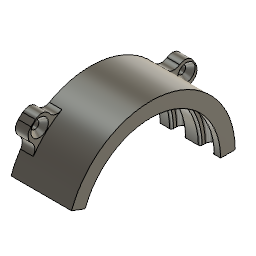
assem_new (Autodesk Fusion 360 archive; units mm, degrees)
design "ring_160"
Autodesk Fusion 360 part; units mm, degrees
note: some values were not read from the file. Chosen so that the rebuilt part matches the saved one: a direction; which face or edge a step refers to. Set by a fixed rule: which sketch regions a step uses.
sketch "Sketch1" plane through (0, 0, 0) normal (0, 0, 1) x (1, 0, 0)
  circle A0 centre (-12.5, 2) radius 1.5
  line L0 (1, -21.5) -> (-17, -21.5)
  line L1 (-17, 0) -> (-17, 5)
  circle A1 centre (-6, 1) radius 1
  line L2 (-17, -21.5) -> (-17, 0)
  line L3 (-14, 2) -> (-14, 1)
  line L4 (-5, 2) -> (-5, 1)
  line L5 (-2, 2) -> (-2, 1)
  circle A2 centre (-15, 1) radius 1
  circle A3 centre (-3.5, 2) radius 1.5
  circle A4 centre (-1, 1) radius 1
  line L6 (1, 0) -> (1, -21.5)
  line L7 (-17, 5) -> (1, 5)
  line L8 (-11, 2) -> (-11, 1)
  line L9 (-17, 0) -> (1, 0)
  circle A5 centre (-10, 1) radius 1
  line L10 (1, 5) -> (1, 0)
  point P0 (-18, 0)
  point P1 (1, 0)
  dimension "d1" = 5
  dimension "d2" = 18
  dimension "d3" = 21.5
  constraint coincident L3.start A0
  constraint coincident L3.end A2
  constraint tangent L3 A2
  constraint coincident L8.start A0
  constraint coincident L8.end A5
  constraint tangent L8 A5
  constraint parallel L3 L8
  constraint coincident L5.start A3
  constraint coincident L5.end A4
  constraint tangent L5 A4
  constraint vertical L5
  constraint coincident L4.start A3
  constraint coincident L4.end A1
  constraint tangent A1 L4
  constraint parallel L4 L5
  constraint horizontal L9
  constraint vertical L6
  constraint horizontal L0
  constraint vertical L2
  measures "d1" distance of L1.start L1.end
  measures "d2" distance of L1.start P1
  measures "d3" distance of L1.start L0.end
revolve "Revolve1" add sketch "Sketch1" angle 160 about axis through (1, -21.5, 0) along (1, 0, 0) contours A0 L1 A1 L3 L4 L5 A2 A3 A4 L7 L8 L9 A5 L10 | A5 | A2 | A1 | A4
move_face "OffsetFaces1" offset -0.2 13 faces at (0.3333, -39.3169, 12.0336) (-1.3717, -38.1094, 13.7645) (-3.0937, -43.9926, 10.7834) (-5.6283, -39.3763, 12.0737) (-7.3333, -39.3169, 12.0336) (-10.3717, -38.1094, 13.7645) (-12.0937, 3.414, 1.2216) (-14.6283, -39.3763, 12.0737) (-16.3333, -41.319, 8.334) (-14, -38.5613, 15.5889) (-5, -18.0303, 22.8488) (-11, -18.0303, 22.8488) (-2, -18.0303, 22.8488)
move_face "OffsetFaces2" offset -0.2 13 faces at (-10.8, -18.0303, 22.8488) (-12.9604, -42.9944, 13.0319) (-10.2973, -41.1191, 9.4058) (-14.2, -42.3462, 9.977) (-7.3333, -41.5034, 8.4115) (-14.7027, -23.5621, 21.6594) (-16.3333, -4.7072, 13.7439) (-0.3333, 0.0959, 2.1228) (-1.2973, -41.1191, 9.4058) (-1.8, -18.0303, 22.8488) (-3.9604, -42.9944, 13.0319) (-5.2, -18.0303, 22.8488) (-5.7027, -11.2033, 19.1666)
sketch "Sketch2" plane through (-17, 0, 0) normal (-1, 0, 0) x (0, -1, 0)
  line L0 (-5, 0) -> (-0.4, 0)
  arc A0 (42.0793, 7.4902) -> (-0.4, 0) centre (21.5, 0) ccw
  line L1 (42.0793, 7.4902) -> (46.4019, 9.0635)
  arc A1 (46.4019, 9.0635) -> (-5, 0) centre (21.5, 0) ccw
  circle A2 centre (21.5, 0) radius 32.5
  line L2 (21.5, 0) -> (-9.04, 11.1157)
  line L3 (21.5, 0) -> (54, 0) construction
  line L4 (21.5, 0) -> (-5.1224, 18.6412)
  line L5 (21.5, 0) -> (54, 0) construction
  line L6 (21.5, 0) -> (-4.6668, 13.6216)
  line L7 (21.5, 0) -> (51, 0) construction
  line L8 (21.5, 0) -> (46.3964, 20.8906)
  line L9 (21.5, 0) -> (54, 0) construction
  line L10 (21.5, 0) -> (40.1412, 26.6224)
  line L11 (21.5, 0) -> (54, 0) construction
  line L12 (21.5, 0) -> (41.4299, 21.7497)
  line L13 (21.5, 0) -> (51, 0) construction
  circle A3 centre (-4.6668, 13.6216) radius 1.25
  circle A4 centre (41.4299, 21.7497) radius 1.25
  dimension "d7" = 65
  dimension "d8" = 160
  dimension "d9" = 145
  dimension "d10" = 152.5
  dimension "d11" = 29.5
  dimension "d12" = 40
  dimension "d13" = 55
  dimension "d14" = 47.5
  dimension "d15" = 29.5
  dimension "d16" = 2.5
  dimension "d17" = 2.5
  dimension "d18" = 32.5
  constraint concentric A0 A2
  constraint horizontal L3
  constraint coincident A0.centre A1.centre
  constraint horizontal L5
  constraint horizontal L7
  constraint horizontal L9
  constraint horizontal L11
  constraint horizontal L13
  constraint coincident L6.end A3.centre
  constraint coincident L12.end A4.centre
  measures "d7" diameter of A2
  measures "d8" angle of L2 L3
  measures "d9" angle of L4 L5
  measures "d10" angle of L6 L7
  measures "d11" distance of A0.centre L6.end
  measures "d12" angle of L8 L9
  measures "d13" angle of L10 L11
  measures "d14" angle of L12 L13
  measures "d15" distance of A0.centre L12.end
  measures "d16" diameter of A3
  measures "d17" diameter of A4
  measures "d18" distance of A0.centre L4.end
extrude "Extrude1" add sketch "Sketch2" against normal blind 3 contours A1 A2 L2 L4 | A1 A2 L8 L10
extrude "Extrude2" add 1 faces at (-17, 0.6845, 12.5418) along direction (-1, 0, 0) blind 1
fillet "Fillet1" radius 3 8 edges at (-16, 0.2075, 15.1998) (-16, 5.1224, 18.6412) (-16, 9.04, 11.1157) (-16, 3.4019, 9.0635) (-16, -36.6998, 21.7075) (-16, -40.1412, 26.6224) (-16, -41.8002, 17.0339) (-16, -46.3964, 20.8906)
chamfer "Chamfer1" distance 1.5 angle 45 2 edges at (-14, 5.8322, 13.1696) (-14, -40.2645, 21.2977)

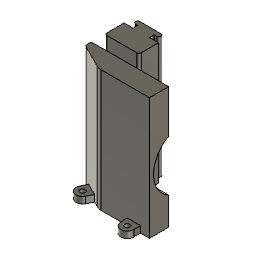
design "vertical_servo_mount"
Autodesk Fusion 360 part; units mm, degrees
sketch "Sketch1" plane through (0, 0, 0) normal (0, 0, 1) x (1, 0, 0)
  line L0 (0, 0) -> (35, 0)
  line L1 (35, 0) -> (35, -25)
  line L2 (35, -25) -> (0, -25)
  line L3 (0, -25) -> (0, 0)
  dimension "d1" = 35
  dimension "d2" = 25
  constraint horizontal L0
  constraint vertical L1
  constraint horizontal L2
  constraint vertical L3
  constraint coincident L0.start L3.end
  measures "d1" distance of L0.start L0.end
  measures "d2" distance of L0.start L2.end
extrude "Extrude1" add sketch "Sketch1" along normal blind 55
sketch "Sketch2" plane through (0, 0, 0) normal (0, 1, 0) x (-1, 0, 0)
  line L0 (-35, 0) -> (0, 0)
  line L1 (0, 0) -> (0, 55)
  line L2 (0, 55) -> (-35, 55)
  line L3 (-35, 55) -> (-35, 0)
  line L4 (-22.7083, 24.0993) -> (-22.7083, 25.6362)
  line L5 (-5.5083, 17.9993) -> (-15.8083, 17.9993)
  line L6 (-5.5083, 18.8493) -> (-0.2083, 18.8493)
  line L7 (-5.5083, 17.9993) -> (-5.5083, 18.8493)
  line L8 (-26.7583, 17.9993) -> (-26.7583, 29.4909)
  line L9 (-15.8083, 14.0493) -> (-15.8083, 13.1993)
  line L10 (-22.7083, 24.0993) -> (-22.7083, 25.6362)
  line L11 (-31.7583, 25.9993) -> (-31.7583, 22.1993)
  line L12 (-15.8083, 44.4493) -> (-15.8083, 14.0493)
  line L13 (-18.3083, 17.9993) -> (-22.5083, 17.9993)
  line L14 (-0.2083, 39.6493) -> (-0.2083, 18.8493)
  line L15 (-15.8083, 18.8493) -> (-15.8083, 17.9993)
  line L16 (-5.5083, 39.6493) -> (-5.5083, 18.8493)
  line L17 (-5.5083, 18.8493) -> (-5.5083, 17.9993)
  line L18 (-30.3583, 22.1993) -> (-30.3583, 25.9993)
  line L19 (-18.3083, 18.8493) -> (-22.5083, 18.8493)
  line L20 (-15.8083, 18.8493) -> (-15.8083, 39.6493)
  line L21 (-15.8083, 14.0493) -> (-18.3083, 14.0493)
  line L22 (-31.7583, 27.5493) -> (-31.7583, 21.8903)
  line L23 (-18.3083, 14.0493) -> (-18.3083, 18.8493)
  line L24 (-0.2083, 17.9993) -> (-5.5083, 17.9993)
  line L25 (-27.9583, 27.5493) -> (-27.9583, 20.6493)
  line L26 (-15.8083, 18.8493) -> (-5.5083, 18.8493)
  line L27 (-5.5083, 18.8493) -> (-5.5083, 39.6493)
  line L28 (-5.5083, 40.4993) -> (-5.5083, 39.6493)
  line L29 (-22.7083, 29.4909) -> (-26.7583, 29.4909)
  line L30 (-0.2083, 39.6493) -> (-5.5083, 39.6493)
  line L31 (-5.5083, 39.6493) -> (-5.5083, 40.4993)
  line L32 (-30.3583, 9.9402) -> (-31.7583, 9.9402)
  line L33 (-31.7583, 40.7256) -> (-30.3583, 40.7256)
  line L34 (-31.7583, 9.9402) -> (-31.7583, 8.0493)
  line L35 (-18.3083, 45.2993) -> (-18.3083, 44.4493)
  line L36 (-22.7083, 22.5625) -> (-22.7083, 24.0993)
  line L37 (-22.7083, 22.5625) -> (-22.7083, 18.1961)
  line L38 (-31.7583, 22.1993) -> (-30.3583, 22.1993)
  line L39 (-31.7583, 25.9993) -> (-30.3583, 25.9993)
  line L40 (-26.7583, 29.4909) -> (-22.7083, 29.4909)
  line L41 (-22.7083, 22.5625) -> (-22.7083, 18.1961)
  line L42 (-22.7083, 17.9993) -> (-22.7083, 18.1961)
  line L43 (-31.7583, 9.9402) -> (-30.3583, 9.9402)
  line L44 (-31.7583, 21.8903) -> (-30.3583, 21.8903)
  line L45 (-31.7583, 25.9993) -> (-31.7583, 40.7256)
  line L46 (-26.7583, 29.6993) -> (-26.7583, 32.4993)
  line L47 (-15.8083, 40.4993) -> (-5.5083, 40.4993)
  line L48 (-30.3583, 22.1993) -> (-31.7583, 22.1993)
  line L49 (-30.3583, 40.7256) -> (-30.3583, 25.9993)
  line L50 (-30.3583, 25.9993) -> (-30.3583, 40.7256)
  line L51 (-31.7583, 40.7256) -> (-31.7583, 25.9993)
  line L52 (-18.3083, 45.2993) -> (-15.8083, 45.2993)
  line L53 (-5.5083, 39.6493) -> (-0.2083, 39.6493)
  line L54 (-18.3083, 39.6493) -> (-18.3083, 44.4493)
  line L55 (-22.7083, 29.4909) -> (-22.7083, 25.6362)
  line L56 (-0.2083, 18.8493) -> (-5.5083, 18.8493)
  line L57 (-18.3083, 18.8493) -> (-18.3083, 17.9993)
  line L58 (-18.3083, 14.0493) -> (-18.3083, 13.1993)
  line L59 (-15.8083, 13.1993) -> (-18.3083, 13.1993)
  line L60 (-22.5083, 18.8493) -> (-22.5083, 22.5373)
  line L61 (-15.8083, 44.4493) -> (-18.3083, 44.4493)
  line L62 (-22.7083, 22.5625) -> (-22.7083, 24.0993)
  line L63 (-22.7083, 17.9993) -> (-22.7083, 18.1961)
  line L64 (-31.7583, 9.9402) -> (-31.7583, 21.8903)
  line L65 (-22.5083, 25.6614) -> (-22.5083, 39.6493)
  line L66 (-30.3583, 21.8903) -> (-31.7583, 21.8903)
  line L67 (-30.3583, 20.6493) -> (-30.3583, 21.8903)
  line L68 (-22.5083, 40.4993) -> (-18.3083, 40.4993)
  line L69 (-0.2083, 40.4993) -> (-0.2083, 39.6493)
  line L70 (-15.8083, 39.6493) -> (-5.5083, 39.6493)
  line L71 (-5.5083, 40.4993) -> (-0.2083, 40.4993)
  line L72 (-15.8083, 40.4993) -> (-15.8083, 39.6493)
  line L73 (-30.3583, 9.9402) -> (-30.3583, 8.0493)
  line L74 (-30.3583, 40.7256) -> (-30.3583, 42.5493)
  line L75 (-15.8083, 45.2993) -> (-15.8083, 44.4493)
  line L76 (-18.3083, 44.4493) -> (-15.8083, 44.4493)
  line L77 (-22.7083, 29.4909) -> (-22.7083, 25.6362)
  line L78 (-5.5083, 39.6493) -> (-15.8083, 39.6493)
  line L79 (-31.7583, 21.8903) -> (-30.3583, 21.8903)
  line L80 (-30.3583, 22.1993) -> (-31.7583, 22.1993)
  line L81 (-31.7583, 25.9993) -> (-30.3583, 25.9993)
  line L82 (-18.3083, 40.4993) -> (-18.3083, 39.6493)
  line L83 (-30.3583, 25.9993) -> (-31.7583, 25.9993)
  line L84 (-22.5083, 17.9993) -> (-22.5083, 18.8493)
  line L85 (-30.3583, 21.8903) -> (-30.3583, 9.9402)
  line L86 (-22.5083, 22.5373) -> (-22.5083, 24.0993)
  line L87 (-22.7083, 32.4993) -> (-22.7083, 29.6993)
  line L88 (-22.7083, 29.6993) -> (-26.7583, 29.6993)
  line L89 (-31.7583, 40.7256) -> (-30.3583, 40.7256)
  line L90 (-22.5083, 39.6493) -> (-22.5083, 40.4993)
  line L91 (-30.3583, 25.9993) -> (-31.7583, 25.9993)
  line L92 (-26.7583, 29.6993) -> (-22.7083, 29.6993)
  line L93 (-22.5083, 39.6493) -> (-18.3083, 39.6493)
  line L94 (-18.3083, 39.6493) -> (-22.5083, 39.6493)
  line L95 (-0.2083, 18.8493) -> (-0.2083, 17.9993)
  line L96 (-30.3583, 9.9402) -> (-31.7583, 9.9402)
  line L97 (-30.3583, 21.8903) -> (-30.3583, 9.9402)
  line L98 (-31.7583, 42.5493) -> (-31.7583, 40.7256)
  line L99 (-30.3583, 40.7256) -> (-31.7583, 40.7256)
  line L100 (-22.5083, 18.8493) -> (-18.3083, 18.8493)
  line L101 (-18.3083, 14.0493) -> (-15.8083, 14.0493)
  line L102 (-5.5083, 18.8493) -> (-15.8083, 18.8493)
  line L103 (-22.5083, 24.0993) -> (-22.5083, 25.6614)
  line L104 (-0.2083, 40.4993) -> (0, 40.4993)
  line L105 (-0.2083, 17.9993) -> (0, 17.9993)
  line L106 (0, 40.4993) -> (-15.6, 40.4993)
  line L107 (-15.6, 40.4993) -> (-15.6, 46.4993)
  line L108 (-15.6, 46.4993) -> (0, 46.4993)
  line L109 (0, 46.4993) -> (0, 40.4993)
  line L110 (0, 17.9993) -> (-15.6, 17.9993)
  line L111 (-15.6, 17.9993) -> (-15.6, 11.9993)
  line L112 (-15.6, 11.9993) -> (0, 11.9993)
  line L113 (0, 11.9993) -> (0, 17.9993)
  line L114 (-15.6, 46.4993) -> (-15.6, 55)
  line L115 (-15.6, 11.9993) -> (-15.6, 0)
  dimension "d5" = 15.6
  dimension "d6" = 6
  dimension "d7" = 15.6
  dimension "d8" = 6
  constraint coincident L1 L104.end
  constraint perpendicular L1 L104
  constraint coincident L1 L105.end
  constraint perpendicular L1 L105
  constraint horizontal L106
  constraint vertical L107
  constraint horizontal L108
  constraint vertical L109
  constraint horizontal L110
  constraint vertical L111
  constraint horizontal L112
  constraint vertical L113
  constraint coincident L2 L114.end
  constraint perpendicular L2 L114
  constraint coincident L0 L115.end
  constraint perpendicular L0 L115
  measures "d5" distance of L104.end L106.end
  measures "d6" distance of L104.end L108.end
  measures "d7" distance of L105.end L110.end
  measures "d8" distance of L105.end L112.end
extrude "Extrude2" cut sketch "Sketch2" against normal blind 12.2 contours L0 L2 L3 L5 L9 L12 L13 L23 L35 L47 L52 L54 L58 L59 L60 L65 L68 L75 L84 L86 L90 L103 L107 L111 L114 L115 | L5 L7 L12 L15 L17 L26 L102 L110 | L1 L14 L69 L95 L104 L105 L106 L110 | L6 L7 L17 L24 L56 L95 L110 | L12 L15 L19 L20 L21 L23 L54 L57 L60 L61 L65 L72 L76 L82 L86 L93 L94 L100 L101 L103 | L6 L14 L16 L27 L30 L53 L56 | L12 L16 L20 L26 L27 L70 L78 L102 | L9 L21 L58 L59 L101 | L35 L52 L61 L75 L76 | L13 L19 L23 L57 L84 L100 | L54 L68 L82 L90 L93 L94 | L11 L18 L22 L38 L39 L48 L80 L81 L83 L91 | L22 L33 L39 L45 L49 L50 L51 L81 L83 L89 L91 L99 | L32 L43 L44 L64 L66 L67 L79 L85 L96 L97
extrude "Extrude3" cut sketch "Sketch2" against normal blind 12.2 contours L12 L28 L31 L47 L70 L72 L78 L106 | L28 L30 L31 L53 L69 L71 L106
sketch "Sketch3" plane through (15.6, 0, 0) normal (1, 0, 0) x (0, 1, 0)
  line L0 (0, 40.4993) -> (0, 55)
  line L1 (0, 55) -> (-12.2, 55)
  line L2 (-12.2, 55) -> (-12.2, 40.4993)
  line L3 (-12.2, 40.4993) -> (0, 40.4993)
  line L4 (-12.2, 40.4993) -> (-6.1, 40.4993)
  line L5 (-6.1, 40.4993) -> (-6.1, 43.1493)
  circle A0 centre (-6.1, 43.1493) radius 0.75
  dimension "d13" = 2.65
  dimension "d14" = 1.5
  constraint coincident L2.end L3.start
  constraint midpoint L3 L4.end
  constraint perpendicular L4 L5
  constraint coincident L5.end A0.centre
  measures "d13" distance of L4.end L5.end
  measures "d14" diameter of A0
extrude "Extrude4" cut sketch "Sketch3" against normal blind 5 contours A0
sketch "Sketch4" plane through (15.6, 0, 0) normal (1, 0, 0) x (0, 1, 0)
  line L0 (0, 0) -> (0, 17.9993)
  line L1 (0, 17.9993) -> (-12.2, 17.9993)
  line L2 (-12.2, 17.9993) -> (-12.2, 0)
  line L3 (-12.2, 0) -> (0, 0)
  line L4 (-12.2, 17.9993) -> (-6.1, 17.9993)
  line L5 (-6.1, 17.9993) -> (-6.1, 15.3493)
  circle A0 centre (-6.1, 15.3493) radius 0.75
  dimension "d17" = 2.65
  dimension "d18" = 1.5
  constraint coincident L1.end L2.start
  constraint midpoint L1 L4.end
  constraint perpendicular L4 L5
  constraint coincident L5.end A0.centre
  measures "d17" distance of L4.end L5.end
  measures "d18" diameter of A0
extrude "Extrude5" cut sketch "Sketch4" against normal blind 5 contours A0
move_face "OffsetFaces1" offset -0.2 1 faces at (5.2, -8.1333, 17.9993)
move_face "OffsetFaces2" offset -0.2 1 faces at (10.4, -8.1333, 40.4993)
move_face "OffsetFaces3" offset -0.1 1 faces at (28.5333, -12.2, 24.2664)
sketch "Sketch5" plane through (15.6, 0, 0) normal (1, 0, 0) x (0, 1, 0)
  circle A0 centre (-6.1, 43.1493) radius 0.75
  line L0 (0, 40.6993) -> (0, 55)
  line L1 (0, 55) -> (-12.3, 55)
  line L2 (-12.3, 55) -> (-12.3, 40.6993)
  line L3 (-12.3, 40.6993) -> (0, 40.6993)
  line L4 (-6.15, 40.6993) -> (-6.15, 17.9993)
  line L5 (-6.15, 40.6993) -> (-6.15, 40.4993)
  line L6 (-6.15, 40.4993) -> (-6.15, 24.0993)
  circle A1 centre (-6.15, 24.0993) radius 12.5
  dimension "d24" = 22.7
  dimension "d25" = 0.2
  dimension "d26" = 16.4
  dimension "d27" = 25
  constraint midpoint L3 L4.start
  constraint perpendicular L3 L4
  constraint perpendicular L3 L5
  constraint parallel L4 L6
  constraint coincident L6.end A1.centre
  measures "d24" distance of L4.start L4.end
  measures "d25" distance of L4.start L5.end
  measures "d26" distance of L5.end L6.end
  measures "d27" diameter of A1
extrude "Extrude6" cut sketch "Sketch5" along normal blind 32 contours A1
move_face "OffsetFaces4" offset -0.5 1 faces at (28.5333, -13.2933, 34.3572)
move_face "OffsetFaces5" offset -4 1 faces at (23.3333, -25, 36.6667)
sketch "Sketch6" plane through (0, 0, 0) normal (0, 1, 0) x (-1, 0, 0)
  line L0 (-15.6, 40.6993) -> (0, 40.6993)
  line L1 (0, 40.6993) -> (0, 55)
  line L2 (0, 55) -> (-15.6, 55)
  line L3 (-15.6, 55) -> (-15.6, 40.6993)
  line L4 (-15.6, 55) -> (0, 55)
  line L5 (0, 55) -> (0, 0)
  line L6 (0, 0) -> (-15.6, 0)
  line L7 (-15.6, 0) -> (-15.6, 55)
  constraint horizontal L4
  constraint vertical L5
  constraint horizontal L6
  constraint vertical L7
  constraint coincident L5.end L6.start
  constraint coincident L2.end L3.start
extrude "Extrude7" add sketch "Sketch6" along normal blind 6.652
move_face "OffsetFaces6" offset -0.1 1 faces at (10.4, 0, 25.4327)
sketch "Sketch7" plane through (0, 0, 0) normal (-1, 0, 0) x (0, -1, 0)
  line L0 (-0.1, 40.6993) -> (12.3, 40.6993)
  line L1 (12.3, 40.6993) -> (12.3, 17.7993)
  line L2 (12.3, 17.7993) -> (-0.1, 17.7993)
  line L3 (-0.1, 17.7993) -> (-0.1, 40.6993)
  line L4 (21, 55) -> (-6.652, 55)
  line L5 (-6.652, 55) -> (-6.652, 0)
  line L6 (-6.652, 0) -> (21, 0)
  line L7 (21, 0) -> (21, 55)
  line L8 (-6.652, 0) -> (-2.552, 0)
  line L9 (-2.552, 0) -> (-2.552, 55)
  line L10 (-2.552, 55) -> (-6.652, 55)
  line L11 (-6.652, 55) -> (-6.652, 0)
  line L12 (-2.552, 55) -> (-4.652, 55)
  line L13 (-4.652, 55) -> (-4.652, 0)
  line L14 (-4.652, 0) -> (-2.552, 0)
  line L15 (-2.552, 0) -> (-2.552, 55)
  dimension "d35" = 4.1
  dimension "d36" = 2.1
  constraint horizontal L8
  constraint vertical L9
  constraint horizontal L10
  constraint vertical L11
  constraint coincident L5.end L6.start
  constraint horizontal L12
  constraint vertical L13
  constraint horizontal L14
  constraint vertical L15
  measures "d35" distance of L5.end L8.end
  measures "d36" distance of L9.end L12.end
extrude "Extrude8" cut sketch "Sketch7" against normal blind 2 contours L4 L5 L6 L8 L10 L11 L13
extrude "Extrude9" cut sketch "Sketch7" against normal blind 4 contours L4 L6 L8 L9 L10 L12 L13 L14 L15
sketch "Sketch8" plane through (15.6, 0, 0) normal (1, 0, 0) x (0, 1, 0)
  circle A0 centre (-6.1, 15.3493) radius 0.75
  circle A1 centre (-6.1, 43.1493) radius 0.75
  line L0 (6.652, 55) -> (-12.3, 55)
  line L1 (-12.3, 55) -> (-12.3, 40.6993)
  line L2 (-12.3, 40.6993) -> (0.1, 40.6993)
  line L3 (0.1, 40.6993) -> (0.1, 17.7993)
  line L4 (0.1, 17.7993) -> (-12.3, 17.7993)
  line L5 (-12.3, 17.7993) -> (-12.3, 35.5526)
  arc A2 (-12.3, 35.5526) -> (-12.3, 12.6461) centre (-6.15, 24.0993) ccw
  line L6 (-12.3, 12.6461) -> (-12.3, 0)
  line L7 (-12.3, 0) -> (6.652, 0)
  line L8 (6.652, 0) -> (6.652, 55)
  line L9 (6.652, 55) -> (2.552, 55)
  line L10 (2.552, 55) -> (2.552, 0)
  line L11 (2.552, 0) -> (6.652, 0)
  line L12 (6.652, 0) -> (6.652, 55)
  line L13 (6.652, 55) -> (4.652, 55)
  line L14 (4.652, 55) -> (4.652, 0)
  line L15 (4.652, 0) -> (6.652, 0)
  line L16 (6.652, 0) -> (6.652, 55)
  dimension "d41" = 4.1
  dimension "d42" = 2
  constraint horizontal L9
  constraint vertical L10
  constraint horizontal L11
  constraint vertical L12
  constraint coincident L0.start L8.end
  constraint horizontal L13
  constraint vertical L14
  constraint horizontal L15
  constraint vertical L16
  measures "d41" distance of L0.start L9.end
  measures "d42" distance of L0.start L13.end
extrude "Extrude10" cut sketch "Sketch8" against normal blind 2 contours L0 L7 L8 L9 L11 L12 L13 L14 L15 L16
extrude "Extrude11" cut sketch "Sketch8" against normal blind 4 contours L0 L7 L9 L10 L11 L14
fillet "Fillet1" radius 1 4 edges at (2, 4.652, 27.5) (2, 6.652, 27.5) (13.6, 4.652, 27.5) (13.6, 6.652, 27.5)
sketch "Sketch9" plane through (0, 0, 0) normal (-1, 0, 0) x (0, -1, 0)
  line L0 (-2.552, 55) -> (-2.552, 0)
  line L1 (-2.552, 0) -> (21, 0)
  line L2 (21, 0) -> (21, 55)
  line L3 (21, 55) -> (-2.552, 55)
  line L4 (-0.1, 40.6993) -> (12.3, 40.6993)
  line L5 (12.3, 40.6993) -> (12.3, 17.7993)
  line L6 (12.3, 17.7993) -> (-0.1, 17.7993)
  line L7 (-0.1, 17.7993) -> (-0.1, 40.6993)
  line L8 (6.1, 17.7993) -> (6.1, 10.7993)
  line L9 (6.1, 10.7993) -> (11.1, 10.7993)
  line L10 (11.1, 10.7993) -> (11.1, 17.7993)
  line L11 (11.1, 17.7993) -> (6.1, 17.7993)
  line L12 (6.1, 17.7993) -> (6.1, 10.7993)
  line L13 (6.1, 10.7993) -> (1.1, 10.7993)
  line L14 (1.1, 10.7993) -> (1.1, 17.7993)
  line L15 (1.1, 17.7993) -> (6.1, 17.7993)
  line L16 (6.1, 17.7993) -> (6.1, 10.7993)
  line L17 (6.1, 17.7993) -> (9.1, 17.7993)
  line L18 (9.1, 17.7993) -> (9.1, 16.7993)
  line L19 (9.1, 16.7993) -> (6.1, 16.7993)
  line L20 (6.1, 16.7993) -> (6.1, 17.7993)
  line L21 (6.1, 16.7993) -> (3.1, 16.7993)
  line L22 (3.1, 16.7993) -> (3.1, 17.7993)
  line L23 (3.1, 17.7993) -> (6.1, 17.7993)
  line L24 (6.1, 17.7993) -> (6.1, 16.7993)
  dimension "d49" = 7
  dimension "d50" = 5
  dimension "d51" = 7
  dimension "d52" = 3
  dimension "d53" = 1
  dimension "d54" = 3
  constraint midpoint L6 L8.start
  constraint perpendicular L6 L8
  constraint horizontal L9
  constraint vertical L10
  constraint horizontal L11
  constraint vertical L12
  constraint horizontal L13
  constraint vertical L14
  constraint horizontal L15
  constraint vertical L16
  constraint horizontal L17
  constraint vertical L18
  constraint horizontal L19
  constraint vertical L20
  constraint horizontal L21
  constraint vertical L22
  constraint horizontal L23
  constraint vertical L24
  measures "d49" distance of L8.start L8.end
  measures "d50" distance of L8.end L9.end
  measures "d51" distance of L8.end L8.start
  measures "d52" distance of L8.start L17.end
  measures "d53" distance of L8.start L19.end
  measures "d54" distance of L19.end L21.end
extrude "Extrude12" cut sketch "Sketch9" against normal blind 10 contours L6 L8 L12 L13 L14 L15 L16 L21 L22 | L6 L8 L9 L10 L11 L12 L16 L18 L19
extrude "Extrude13" cut 1 faces at (0, -7.1, 17.1327) along direction (1, 0, 0) blind 10
extrude "Extrude14" cut sketch "Sketch9" against normal blind 23 contours L6 L8 L12 L15 L16 L20 L21 L22 L23 L24 | L6 L8 L11 L12 L16 L17 L18 L19 L20 L24
fillet "Fillet2" radius 1 4 edges at (12.8, -3.1, 16.7993) (12.8, -3.1, 17.7993) (12.8, -9.1, 17.7993) (12.8, -9.1, 16.7993)
move_face "OffsetFaces7" offset -0.1 2 faces at (11.6, 3.252, 18.3333) (4, 3.952, 18.3333)
sketch "Sketch10" plane through (0, 0, 55) normal (0, 0, 1) x (-1, 0, 0)
  arc A0 (-12.6, -4.652) -> (-12.6, -6.652) centre (-12.6, -5.652) ccw
  line L0 (-12.6, -6.652) -> (-3, -6.652)
  arc A1 (-3, -6.652) -> (-3, -4.652) centre (-3, -5.652) ccw
  line L1 (-3, -4.652) -> (-4.1, -4.652)
  line L2 (-4.1, -4.652) -> (-4.1, -2.552)
  line L3 (-4.1, -2.552) -> (0, -2.552)
  line L4 (0, -2.552) -> (0, 21)
  line L5 (0, 21) -> (-35, 21)
  line L6 (-35, 21) -> (-35, 12.3)
  line L7 (-35, 12.3) -> (-15.6, 12.3)
  line L8 (-15.6, 12.3) -> (-15.6, -2.552)
  line L9 (-15.6, -2.552) -> (-11.5, -2.552)
  line L10 (-11.5, -2.552) -> (-11.5, -4.652)
  line L11 (-11.5, -4.652) -> (-12.6, -4.652)
  line L12 (-15.6, 12.3) -> (0, 12.3)
  line L13 (0, 12.3) -> (0, 6.3)
  line L14 (0, 6.3) -> (-15.6, 6.3)
  line L15 (-15.6, 6.3) -> (-15.6, 12.3)
  dimension "d64" = 6
  constraint horizontal L12
  constraint vertical L13
  constraint horizontal L14
  constraint vertical L15
  constraint coincident L7.end L8.start
  measures "d64" distance of L7.end L14.end
extrude "Extrude15" cut sketch "Sketch10" against normal blind 10 contours L4 L8 L12 L13 L14 L15
fillet "Fillet3" radius 1 5 edges at (15.6, -9.3, 45) (15.6, -6.3, 50) (0, -12.3, 50) (0, -6.3, 50) (0, -9.3, 45)
sketch "Sketch11" plane through (0, 0, 55) normal (0, 0, 1) x (-1, 0, 0)
  arc A0 (-1, 12.3) -> (0, 13.3) centre (-1, 13.3) ccw
  line L0 (0, 13.3) -> (0, 21)
  line L1 (0, 21) -> (-35, 21)
  line L2 (-35, 21) -> (-35, 12.3)
  line L3 (-35, 12.3) -> (-1, 12.3)
  line L4 (0, 21) -> (0, 15)
  line L5 (0, 21) -> (-12, 21)
  line L6 (0, 15) -> (-12, 21)
  dimension "d69" = 12
  constraint coincident L0.end L1.start
  constraint coincident L0 L4.end
  constraint perpendicular L4 L5
  measures "d69" distance of L0.end L5.end
extrude "Extrude16" cut sketch "Sketch11" against normal blind 100 contours L0 L1 L4 L5 L6
fillet "Fillet4" radius 1.5 1 edges at (0, -15, 27.5)
fillet "Fillet5" radius 5 1 edges at (12, -21, 27.5)
sketch "Sketch12" plane through (0, 0, 0) normal (0, 0, -1) x (1, 0, 0)
  arc A0 (13.1803, 21) -> (10.9443, 20.4721) centre (13.1803, 16) ccw
  line L0 (10.9443, 20.4721) -> (0.8292, 15.4146)
  arc A1 (0.8292, 15.4146) -> (0, 14.0729) centre (1.5, 14.0729) ccw
  line L1 (0, 14.0729) -> (0, -2.552)
  line L2 (0, -2.552) -> (4.1, -2.552)
  line L3 (4.1, -2.552) -> (4.1, -4.652)
  line L4 (4.1, -4.652) -> (3, -4.652)
  arc A2 (3, -4.652) -> (3, -6.652) centre (3, -5.652) ccw
  line L5 (3, -6.652) -> (12.6, -6.652)
  arc A3 (12.6, -6.652) -> (12.6, -4.652) centre (12.6, -5.652) ccw
  line L6 (12.6, -4.652) -> (11.5, -4.652)
  line L7 (11.5, -4.652) -> (11.5, -2.552)
  line L8 (11.5, -2.552) -> (15.6, -2.552)
  line L9 (15.6, -2.552) -> (15.6, 12.3)
  line L10 (15.6, 12.3) -> (35, 12.3)
  line L11 (35, 12.3) -> (35, 21)
  line L12 (35, 21) -> (13.1803, 21)
  line L13 (35, 21) -> (31, 21)
  line L14 (31, 21) -> (25, 21)
  line L15 (25, 21) -> (25, 27)
  line L16 (25, 27) -> (31, 27)
  line L17 (31, 27) -> (31, 21)
  circle A4 centre (28, 24) radius 1.15
  circle A5 centre (28, 24) radius 3
  line L18 (0, -2.552) -> (0, 1.448)
  line L19 (0, 1.448) -> (-6, 1.448)
  line L20 (-6, 1.448) -> (-6, 7.448)
  line L21 (-6, 7.448) -> (0, 7.448)
  line L22 (0, 7.448) -> (0, 1.448)
  circle A6 centre (-3, 4.448) radius 1.15
  circle A7 centre (-3, 4.448) radius 3
  line L23 (0.8292, 15.4146) -> (3.0652, 16.5326)
  line L24 (3.0652, 16.5326) -> (8.4318, 19.2159)
  line L25 (3.0652, 16.5326) -> (0.382, 21.8992)
  line L26 (1.7236, 19.2159) -> (4.4069, 20.5575)
  circle A8 centre (4.4069, 20.5575) radius 1.15
  circle A9 centre (4.4069, 20.5575) radius 3
  line L27 (8.4318, 19.2159) -> (7.0902, 21.8992)
  dimension "d76" = 6
  dimension "d77" = 2.3
  dimension "d78" = 4
  dimension "d79" = 6
  dimension "d80" = 6
  dimension "d81" = 2.3
  dimension "d82" = 2.5
  dimension "d83" = 6
  dimension "d84" = 6
  dimension "d85" = 3
  dimension "d86" = 2.3
  constraint coincident L11.end L12.start
  constraint coincident L12 L13.end
  constraint horizontal L14
  constraint vertical L15
  constraint horizontal L16
  constraint vertical L17
  constraint concentric A4 A5
  constraint tangent L17 A5
  constraint coincident L1.end L2.start
  constraint perpendicular L2 L18
  constraint horizontal L19
  constraint vertical L20
  constraint horizontal L21
  constraint vertical L22
  constraint concentric A6 A7
  constraint tangent L21 A7
  constraint coincident L0.end A1.start
  constraint parallel L0 L23
  constraint parallel L0 L24
  constraint perpendicular L24 L25
  constraint midpoint L25 L26.start
  constraint perpendicular L25 L26
  constraint coincident L26.end A8.centre
  constraint coincident L26.start A9
  constraint coincident A9 L27.end
  constraint tangent A9 L27
  measures "d76" distance of L13.end L14.end
  measures "d77" diameter of A4
  measures "d78" distance of L1.end L18.end
  measures "d79" distance of L18.end L19.end
  measures "d80" distance of L18.end L21.end
  measures "d81" diameter of A6
  measures "d82" distance of L0.end L23.end
  measures "d83" distance of L23.end L24.end
  measures "d84" distance of L23.end L25.end
  measures "d85" distance of L26.start L26.end
  measures "d86" diameter of A8
extrude "Extrude17" add sketch "Sketch12" against normal blind 3 contours L12 L14 L15 A5 | L0 L24 A9 L27 | L12 L14 L17 A5 | A5 | L0 L24 L25 A9 | A9 | L1 L21 L22 A7 | A7 | L1 L19 L22 A7
